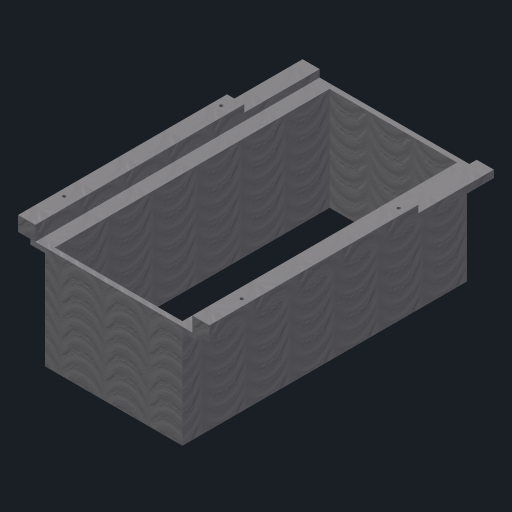
# Autodesk Inventor part: PUERTA_ACOPLE_ENTRADA
Saved by Autodesk Inventor 2024.3 (Build 283343000, 343)
## iProperties
Created: 2024-07-11
Part Number: PUERTA_ACOPLE_ENTRADA
Material: Steel, Mild, Welded
Document SubType Name: Modeling
Designer: Niler
Density: 7.85 g/cm^3
Appearance: Weld - Steel Mild
Author: Niler
Autodesk Inventor part; units mm, degrees
ref_plane "YZ Plane" through (0, 0, 0) normal (1, 0, 0) x (0, 1, 0)
ref_plane "XZ Plane" through (0, 0, 0) normal (0, 1, 0) x (-1, 0, 0)
ref_plane "XY Plane" through (0, 0, 0) normal (0, 0, 1) x (1, 0, 0)
sketch "Sketch1" plane through (0, 0, 0) normal (0, 1, 0) x (-1, 0, 0)
  line L0 (-90.5, 80) -> (90.5, 80) construction
  line L1 (90.5, 80) -> (90.5, -80) construction
  line L2 (90.5, -80) -> (-90.5, -80) construction
  line L3 (-90.5, -80) -> (-90.5, 80) construction
  line L4 (-90.5, 80) -> (90.5, -80) construction
  line L5 (90.5, 80) -> (-90.5, -80) construction
  circle A0 centre (90.5, 80) radius 1.65
  circle A1 centre (90.5, -80) radius 1.65
  circle A2 centre (-90.5, -80) radius 1.65
  circle A3 centre (-90.5, 80) radius 1.65
  line L6 (97.5, 120) -> (-97.5, 120)
  line L7 (-97.5, 120) -> (-97.5, -170)
  line L8 (-97.5, -170) -> (97.5, -170)
  line L9 (97.5, -170) -> (97.5, 120)
  line L10 (80, 120) -> (80, -170)
  line L11 (0, 0) -> (0, -42.6616)
  line L12 (-80, 120) -> (-80, -170)
  line L13 (-97.5, -93) -> (97.5, -93)
  point P0 (0, -170)
  point P1 (-80, -93)
  point P2 (80, -93)
  dimension "d0" = 181
  dimension "d1" = 160
  dimension "d2" = 3.3
  dimension "d3" = 40
  dimension "d4" = 290
  dimension "d5" = 7
  dimension "d7" = 10.5
  dimension "d8" = 13
  constraints: 28 end point, 4 centre point, 4 coincident, 4 parallel, 4 perpendicular, 4 point on line, 3 equal radius, 3 midpoint, 2 horizontal, 2 symmetric about line, 1 vertical, 1 vertical alignment
  measures "d0" distance of L1.end L2.end
  measures "d1" distance of L0.end L1.end
  measures "d2" diameter of A0
  measures "d3" distance from line of A0.centre L6
  measures "d4" distance of L8.end L6.start
  measures "d5" distance between parallel lines of L1 L9
  measures "d7" distance from line of L10 A0.centre
  measures "d8" distance from line of L13 A2.centre
extrude "Extrusion1" add sketch "Sketch1" along normal blind 7.5 contours L9 L13 L10 L6 | L12 L13 L7 L6
extrude "Extrusion2" add sketch "Sketch1" against normal blind 7.5 contours L9 L13 L10 L6 | L9 L8 L10 L13 | L12 L13 L7 L6 | L12 L8 L7 L13
sketch "Sketch2" plane through (0, -7.5, 0) normal (0, -1, 0) x (1, 0, 0)
  line L0 (97.5, 120) -> (80, 120) projected
  line L1 (80, 120) -> (80, -170) projected
  line L2 (80, -170) -> (97.5, -170) projected
  line L3 (97.5, -170) -> (97.5, 120) projected
  circle A0 centre (90.5, 80) radius 1.65 projected
  circle A1 centre (90.5, -80) radius 1.65 projected
  line L4 (-97.5, -170) -> (-80, -170) projected
  line L5 (-80, -170) -> (-80, 120) projected
  line L6 (-80, 120) -> (-97.5, 120) projected
  line L7 (-97.5, 120) -> (-97.5, -170) projected
  circle A2 centre (-90.5, -80) radius 1.65 projected
  circle A3 centre (-90.5, 80) radius 1.65 projected
  line L8 (-80, -170) -> (80, -170)
  line L9 (80, -170) -> (80, 120)
  line L10 (80, 120) -> (-80, 120)
  line L11 (-80, 120) -> (-80, -170)
  line L12 (-80, -170) -> (-85, -170)
  line L13 (-85, -170) -> (-85, 120)
  line L14 (-85, 120) -> (-80, 120)
  line L15 (-80, 120) -> (-80, -170)
  line L16 (-70, -170) -> (70, -170)
  line L17 (70, -170) -> (70, 120)
  line L18 (70, 120) -> (-70, 120)
  line L19 (-70, 120) -> (-70, -170)
  line L20 (0, 0) -> (0, 25.7768)
  line L21 (85, -170) -> (85, 120)
  point P0 (0, 120)
  point P1 (85, 120)
  dimension "d13" = 5
  dimension "d14" = 140
  constraints: 28 end point, 6 parallel, 3 horizontal, 3 perpendicular, 3 point on line, 2 midpoint, 2 symmetric about line, 1 vertical
  measures "d13" distance between parallel lines of L5 L13
  measures "d14" distance between parallel lines of L17 L19
extrude "Extrusion3" add sketch "Sketch2" along normal blind 5 contours L21 L2 L1 L0 | L1 L8 L17 L10 | L19 L8 L5 L10 | L5 L4 L13 L6
sketch "Sketch3" plane through (0, -12.5, 0) normal (0, -1, 0) x (1, 0, 0)
  line L0 (-85, -170) -> (-70, -170) projected
  line L1 (-70, -170) -> (-70, 120) projected
  line L2 (-70, 120) -> (-85, 120) projected
  line L3 (-85, 120) -> (-85, -170) projected
  line L4 (85, 120) -> (70, 120) projected
  line L5 (70, 120) -> (70, -170) projected
  line L6 (70, -170) -> (85, -170) projected
  line L7 (85, -170) -> (85, 120) projected
  line L8 (-70, -170) -> (70, -170)
  line L9 (70, -170) -> (70, 120)
  line L10 (70, 120) -> (-70, 120)
  line L11 (-70, 120) -> (-70, -170)
  line L12 (65, -165) -> (-65, -165)
  line L13 (-65, -165) -> (-65, 115)
  line L14 (-65, 115) -> (65, 115)
  line L15 (65, 115) -> (65, -165)
  point P0 (0, 0)
  dimension "d19" = 140
  dimension "d20" = 290
  dimension "d21" = 5
  constraints: 16 end point, 4 parallel, 2 perpendicular, 1 horizontal, 3 other
  measures "d19" distance of L10.end L9.end
  measures "d20" distance of L9.end L8.end
  measures "d21" distance between parallel lines of L8 L12
extrude "Extrusion4" add sketch "Sketch3" along normal blind 100 and the other way blind 5 contours L1 L10 L5 L8
body "Solid1"
